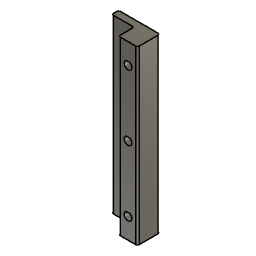
IKEA Trofast Bin to drawer bracket (Autodesk Fusion 360 design; units mm, degrees)
Autodesk Fusion 360 part; units mm, degrees
sketch "Sketch1" plane through (0, 0, 0) normal (0, 0, 1) x (1, 0, 0)
  line L0 (0, 0) -> (-24, 0)
  line L1 (-24, 0) -> (-24, -4)
  line L2 (-24, -4) -> (-11, -4)
  line L3 (-11, -4) -> (-11, -13)
  line L4 (-11, -13) -> (0, -13)
  line L5 (0, -13) -> (0, 0)
  dimension "d1" = 4
  dimension "d2" = 13
  dimension "d3" = 11
  dimension "d4" = 9
  constraint coincident L0.start L5.end
  constraint horizontal L0
  constraint perpendicular L0 L1
  constraint perpendicular L1 L2
  constraint perpendicular L0 L3
  constraint perpendicular L1 L4
  constraint perpendicular L0 L5
  measures "d1" distance of L0.end L1.end
  measures "d2" distance of L1.end L3
  measures "d3" distance of L3.end L4.end
  measures "d4" vertical distance of L1.end L3.end
extrude "Extrude1" add sketch "Sketch1" along normal blind 100
sketch "Sketch2" plane through (0, 0, 0) normal (0, 1, 0) x (-1, 0, 0)
  line L0 (0, 0) -> (24, 0)
  line L1 (24, 0) -> (24, 100)
  line L2 (24, 100) -> (0, 100)
  line L3 (0, 100) -> (0, 0)
  line L4 (0, 0) -> (0, 100)
  line L5 (11, 0) -> (11, 100)
  line L6 (11, 100) -> (0, 100)
  line L7 (11, 0) -> (0, 0)
  line L8 (5.5, 100) -> (5.5, 0) construction
  line L9 (5.5, 14.2479) -> (5.5, 13.9479) construction
  line L10 (6.6219, 13.9479) -> (4.3781, 13.9479)
  arc A0 (4.3781, 13.9479) -> (6.6219, 13.9479) centre (5.5, 12) ccw
  arc A1 (6.6219, 13.9479) -> (5.5, 14.2479) centre (5.5, 12) ccw construction
  arc A2 (5.5, 14.2479) -> (4.3781, 13.9479) centre (5.5, 12) ccw construction
  dimension "d8" = 0.3
  dimension "d10" = 12
  dimension "d11" = 4.4958
  constraint midpoint L6 L8.start
  constraint midpoint L7 L8.end
  constraint coincident L8 A0.centre
  constraint coincident L8 L9.start
  constraint coincident L8 L9.end
  constraint horizontal L10
  constraint coincident L9.end L10
  constraint concentric A0 A1
  constraint concentric A0 A2
  measures "d8" distance of L9.start L9.end
  measures "d10" distance of L8.end A0.centre
  measures "d11" diameter of A0
extrude "Extrude2" cut sketch "Sketch2" against normal blind 13 contours L10 A0
pattern_linear "R-Pattern1" count 3 spacing 38 along (0, 0, 1) of "Extrude2"
fillet "Fillet1" radius 1 6 edges at (0, 0, 50) (-24, 0, 50) (-24, -4, 50) (-11, -4, 50) (-11, -13, 50) (0, -13, 50)
named bodies: "IKEA Trofast Bin to drawer bracket"
